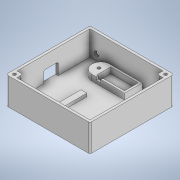
# Autodesk Inventor part: caixa box
Saved by Autodesk Inventor 2022 (Build 260153000, 153)
## iProperties
Created: 2022-04-15
Part Number: caixa box
Material: Genérico
Document SubType Name: Modeling
Designer: Hanter
Density: 1 g/cm^3
Appearance: Padrão
Author: Hanter
Autodesk Inventor part; units mm, degrees
ref_plane "YZ Plane" through (0, 0, 0) normal (1, 0, 0) x (0, 1, 0)
ref_plane "XZ Plane" through (0, 0, 0) normal (0, 1, 0) x (-1, 0, 0)
ref_plane "XY Plane" through (0, 0, 0) normal (0, 0, 1) x (1, 0, 0)
sketch "Esboço1" plane through (0, 0, 0) normal (0, 1, 0) x (-1, 0, 0)
  line L0 (-40, 40) -> (40, 40)
  line L1 (40, 40) -> (40, -40)
  line L2 (40, -40) -> (-40, -40)
  line L3 (-40, -40) -> (-40, 40)
  line L4 (-40, 40) -> (40, -40) construction
  line L5 (40, 40) -> (-40, -40) construction
  point P0 (0, 0)
  dimension "d0" = 80
  dimension "d1" = 80
  constraints: 12 end point, 2 midpoint, 2 parallel, 1 horizontal, 1 perpendicular
  measures "d0" distance of L1.end L2.end
  measures "d1" distance of L0.end L1.end
extrude "Extrusão1" add sketch "Esboço1" along normal blind 2.5
sketch "Esboço2" plane through (0, 2.5, 0) normal (0, 1, 0) x (1, 0, 0)
  circle A0 centre (33, -28) radius 1.5875
  line L0 (-40, -40) -> (40, -40) projected
  line L1 (40, -40) -> (40, 40) projected
  circle A1 centre (33, -0.06) radius 1.5875
  circle A2 centre (33, -28) radius 4.5
  circle A3 centre (33, -0.06) radius 4.5
  dimension "d4" = 3.175
  dimension "d5" = 12
  dimension "d6" = 7
  dimension "d7" = 3.175
  dimension "d8" = 27.94
  dimension "d9" = 9
  dimension "d10" = 9
  constraints: 4 centre point, 2 coincident
  measures "d4" diameter of A0
  measures "d5" distance from line of L0 A0.centre
  measures "d6" distance from line of L1 A0.centre
  measures "d7" diameter of A1
  measures "d8" distance of A1.centre A0.centre
  measures "d9" diameter of A3
  measures "d10" diameter of A2
extrude "Extrusão2" add sketch "Esboço2" along normal blind 3
sketch "Esboço3" plane through (0, 2.5, 0) normal (0, 1, 0) x (1, 0, 0)
  line L0 (-6.9727, -23.0834) -> (-13.0273, -23.0834)
  line L1 (-13.0273, -23.0834) -> (-13.0273, 3.9103)
  line L2 (-13.0273, 3.9103) -> (-6.9727, 3.9103)
  line L3 (-6.9727, 3.9103) -> (-6.9727, -23.0834)
  line L4 (-6.9727, -23.0834) -> (-13.0273, 3.9103) construction
  line L5 (-13.0273, -23.0834) -> (-6.9727, 3.9103) construction
  line L6 (40, -40) -> (40, 40) projected
  point P0 (0, 0)
  point P1 (-10, -9.5866)
  dimension "d13" = 50
  constraints: 12 end point, 2 midpoint, 2 parallel, 1 horizontal, 1 perpendicular
  measures "d13" distance from line of L6 point (-10, -9.587)
extrude "Extrusão3" add sketch "Esboço3" along normal blind 3
sketch "Esboço4" plane through (0, 2.5, 0) normal (0, 1, 0) x (1, 0, 0)
  line L0 (13, 36) -> (-15, 36)
  line L1 (-15, 36) -> (-15, 22)
  line L2 (-15, 22) -> (13, 22)
  line L3 (13, 22) -> (13, 36)
  line L4 (35.54, 17.72) -> (-33.04, 17.72)
  line L5 (-33.04, 17.72) -> (-33.04, -35.62)
  line L6 (-33.04, -35.62) -> (35.54, -35.62)
  line L7 (35.54, -35.62) -> (35.54, 17.72)
  circle A0 centre (33, -28) radius 1.5875 projected
  line L8 (15, 38) -> (-17, 38)
  line L9 (-17, 38) -> (-17, 20)
  line L10 (-17, 20) -> (15, 20)
  line L11 (15, 20) -> (15, 38)
  line L12 (40, 40) -> (-40, 40) projected
  line L13 (40, -40) -> (40, 40) projected
  point P0 (0, 0)
  dimension "d16" = 28
  dimension "d17" = 14
  dimension "d18" = 68.58
  dimension "d19" = 53.34
  dimension "d20" = 7.62
  dimension "d21" = 2.54
  dimension "d22" = 4
  dimension "d23" = 27
  dimension "d24" = 2
  dimension "d25" = 2
  dimension "d26" = 2
  dimension "d27" = 2
  constraints: 24 end point, 6 parallel, 3 horizontal, 3 perpendicular
  measures "d16" distance of L2.end L1.end
  measures "d17" distance of L1.end L0.end
  measures "d18" distance of L6.end L5.end
  measures "d19" distance of L5.end L4.end
  measures "d20" distance from line of L6 A0.centre
  measures "d21" distance from line of L7 A0.centre
  measures "d22" distance between parallel lines of L12 L0
  measures "d23" distance between parallel lines of L13 L3
  measures "d24" distance between parallel lines of L8 L0
  measures "d25" distance between parallel lines of L9 L1
  measures "d26" distance between parallel lines of L10 L2
  measures "d27" distance between parallel lines of L11 L3
extrude "Extrusão4" add sketch "Esboço4" along normal blind 6 contours L11 L10 L9 L8
sketch "Esboço5" plane through (-17, 2.5, -20) normal (0, 0, 1) x (1, 0, 0)
  line L0 (0, 6) -> (32, 6) projected
  line L1 (3.1604, 6) -> (8.0765, 6)
  line L2 (8.0765, 6) -> (8.0765, 3)
  line L3 (8.0765, 3) -> (3.1604, 3)
  line L4 (3.1604, 3) -> (3.1604, 6)
  point P0 (17, -2.5)
  dimension "d32" = 3
  constraints: 8 end point, 2 parallel, 1 horizontal, 1 perpendicular, 1 point on line
  measures "d32" distance between parallel lines of L0 L3
extrude "Extrusão5" cut sketch "Esboço5" against normal blind 6
sketch "Esboço6" plane through (0, 2.5, 0) normal (0, 1, 0) x (1, 0, 0)
  line L0 (15, 20) -> (-17, 20) projected
  line L1 (-17, 20) -> (-27, 20)
  line L2 (-27, 20) -> (-27, 38)
  line L3 (-27, 38) -> (-17, 38)
  line L4 (-17, 38) -> (-17, 20)
  point P0 (0, 0)
  dimension "d33" = 10
  constraints: 8 end point, 2 parallel, 1 horizontal, 1 perpendicular
  measures "d33" distance of L2.end L3.end
extrude "Extrusão6" add sketch "Esboço6" along normal blind 6
fillet "Arredondamento1" radius 9 2 edges at (-27, 5.5, -20) (-27, 5.5, -38)
sketch "Esboço7" plane through (0, 8.5, 0) normal (0, 1, 0) x (1, 0, 0)
  circle A0 centre (-19.962, 29) radius 1.5
  point P0 (0, 0)
  dimension "d37" = 3
  constraints: 1 centre point
  measures "d37" diameter of A0
extrude "Extrusão7" cut sketch "Esboço7" against normal blind 6
sketch "Esboço8" plane through (0, 2.5, 0) normal (0, 1, 0) x (1, 0, 0)
  line L0 (-42.5, -42.5) -> (42.5, -42.5)
  line L1 (42.5, -42.5) -> (42.5, 42.5)
  line L2 (42.5, 42.5) -> (-42.5, 42.5)
  line L3 (-42.5, 42.5) -> (-42.5, -42.5)
  line L4 (40, 40) -> (-40, 40) projected
  line L5 (-40, 40) -> (-40, -40) projected
  line L6 (-40, -40) -> (40, -40) projected
  line L7 (40, -40) -> (40, 40) projected
  point P0 (0, 0)
  dimension "d40" = 2.5
  dimension "d41" = 2.5
  dimension "d42" = 2.5
  dimension "d43" = 2.5
  constraints: 8 end point, 2 parallel, 1 horizontal, 1 perpendicular
  measures "d40" distance between parallel lines of L2 L4
  measures "d41" distance between parallel lines of L3 L5
  measures "d42" distance between parallel lines of L0 L6
  measures "d43" distance between parallel lines of L1 L7
extrude "Extrusão8" add sketch "Esboço8" along normal blind 25 and the other way blind 2.5
fillet "Arredondamento2" radius 2 4 edges at (-42.5, 13.75, 42.5) (-42.5, 13.75, -42.5) (42.5, 13.75, 42.5) (42.5, 13.75, -42.5)
sketch "Esboço10" plane through (-42.5, 0, -40.5) normal (-1, 0, 0) x (0, 0, 1)
  line L0 (76.52, 0) -> (23.18, 0)
  line L1 (81, 27.5) -> (81, 0) projected
  line L2 (0.5, 2.5) -> (80.5, 2.5) projected
  line L3 (32.58, 2.5) -> (47.58, 2.5)
  line L4 (47.58, 2.5) -> (47.58, 14.5)
  line L5 (47.58, 14.5) -> (32.58, 14.5)
  line L6 (32.58, 14.5) -> (32.58, 2.5)
  point P0 (40.5, 0)
  dimension "d51" = 15
  dimension "d52" = 12
  constraints: 10 end point, 2 horizontal, 2 parallel, 1 perpendicular, 1 point on line
  measures "d51" distance of L5.end L4.end
  measures "d52" distance of L4.end L3.end
extrude "Extrusão9" cut sketch "Esboço10" against normal blind 3
fillet "Arredondamento3" radius 2 2 edges at (-41.25, 14.5, 7.08) (-41.25, 14.5, -7.92)
sketch "Esboço11" plane through (0, 27.5, 0) normal (0, 1, 0) x (1, 0, 0)
  line L0 (40, -40) -> (40, 40) projected
  line L1 (40, 40) -> (34, 40)
  line L2 (34, 40) -> (34, 34)
  line L3 (34, 34) -> (40, 34)
  line L4 (40, 34) -> (40, 40)
  line L5 (-40, -7.08) -> (-40, -40) projected
  line L6 (-40, -40) -> (-34, -40)
  line L7 (-34, -40) -> (-34, -34)
  line L8 (-34, -34) -> (-40, -34)
  line L9 (-40, -34) -> (-40, -40)
  point P0 (0, 0)
  dimension "d57" = 6
  dimension "d58" = 6
  dimension "d59" = 6
  dimension "d60" = 6
  constraints: 16 end point, 4 parallel, 2 horizontal, 2 perpendicular
  measures "d57" distance of L3.end L2.end
  measures "d58" distance of L2.end L1.end
  measures "d59" distance of L8.end L7.end
  measures "d60" distance of L7.end L6.end
extrude "Extrusão10" add sketch "Esboço11" against normal blind 25
fillet "Arredondamento4" radius 2 2 edges at (-34, 15, 34) (34, 15, -34)
sketch "Esboço12" plane through (0, 27.5, 0) normal (0, 1, 0) x (1, 0, 0)
  circle A0 centre (-38.25, -38.25) radius 1.5
  circle A1 centre (38.25, 38.25) radius 1.5
  line L0 (40.5, 42.5) -> (-40.5, 42.5) projected
  line L1 (42.5, -40.5) -> (42.5, 40.5) projected
  line L2 (-40.5, -42.5) -> (40.5, -42.5) projected
  line L3 (-42.5, 40.5) -> (-42.5, -40.5) projected
  point P0 (0, 0)
  dimension "d64" = 3
  dimension "d65" = 3
  dimension "d66" = 4.25
  dimension "d67" = 4.25
  dimension "d68" = 4.25
  dimension "d69" = 4.25
  constraints: 2 centre point
  measures "d64" diameter of A0
  measures "d65" diameter of A1
  measures "d66" distance from line of L0 A1.centre
  measures "d67" distance from line of L1 A1.centre
  measures "d68" distance from line of L2 A0.centre
  measures "d69" distance from line of L3 A0.centre
extrude "Extrusão11" cut sketch "Esboço12" against normal blind 10
sketch "Esboço13" plane through (40.5, 0, -42.5) normal (0, 0, -1) x (-1, 0, 0)
  circle A0 centre (73.7947, 8.7851) radius 2.5
  point P0 (40.5, 0)
  dimension "d72" = 5
  constraints: 1 centre point
  measures "d72" diameter of A0
extrude "Extrusão12" cut sketch "Esboço13" against normal blind 10
